Autodesk Inventor part; units mm, degrees
(part 3 of 3)
sketch "Sketch13" plane through (0, 0, 20) normal (0, 0, 1) x (1, 0, 0)
  arc A0 (68.9429, -68.9429) -> (69.4823, -68.3993) centre (0, 0) ccw projected
  arc A1 (69.4823, -68.3993) -> (73.8041, -70.4056) centre (83.4681, -43.9299) ccw projected
  arc A2 (73.8041, -70.4056) -> (74.9009, -69.2377) centre (0, 0) ccw projected
  arc A3 (74.9009, -69.2377) -> (72.6272, -65.0503) centre (49.0843, -80.5451) ccw projected
  arc A4 (72.6272, -65.0503) -> (73.64, -63.9015) centre (0, 0) ccw projected
  arc A5 (73.64, -63.9015) -> (78.0793, -65.6325) centre (86.0618, -38.6023) ccw projected
  arc A6 (78.0793, -65.6325) -> (79.1006, -64.398) centre (0, 0) ccw projected
  arc A7 (79.1006, -64.398) -> (76.5684, -60.3617) centre (54.0449, -77.3041) ccw projected
  arc A8 (76.5684, -60.3617) -> (77.5071, -59.1515) centre (0, 0) ccw projected
  arc A9 (77.5071, -59.1515) -> (82.0463, -60.6003) centre (88.3159, -33.1222) ccw projected
  arc A10 (82.0463, -60.6003) -> (82.9881, -59.3041) centre (0, 0) ccw projected
  arc A11 (82.9881, -59.3041) -> (80.2075, -55.4348) centre (58.7922, -73.758) ccw projected
  arc A12 (80.2075, -55.4348) -> (81.0683, -54.1681) centre (0, 0) ccw projected
  arc A13 (81.0683, -54.1681) -> (85.6895, -55.329) centre (90.2213, -27.5115) ccw projected
  arc A14 (85.6895, -55.329) -> (86.548, -53.9763) centre (0, 0) ccw projected
  arc A15 (86.548, -53.9763) -> (83.53, -50.2891) centre (63.3075, -69.9209) ccw projected
  arc A16 (83.53, -50.2891) -> (84.3096, -48.9709) centre (0, 0) ccw projected
  arc A17 (84.3096, -48.9709) -> (88.9946, -49.8394) centre (91.7708, -21.7921) ccw projected
  arc A18 (88.9946, -49.8394) -> (89.7665, -48.4354) centre (0, 0) ccw projected
  arc A19 (89.7665, -48.4354) -> (86.5228, -44.945) centre (67.5729, -65.8078) ccw projected
  arc A20 (86.5228, -44.945) -> (87.2181, -43.5804) centre (0, 0) ccw projected
  arc A21 (87.2181, -43.5804) -> (91.9484, -44.153) centre (92.958, -15.9868) ccw projected
  arc A22 (91.9484, -44.153) -> (92.6306, -42.7033) centre (0, 0) ccw projected
  arc A23 (92.6306, -42.7033) -> (89.1742, -39.4235) centre (71.5717, -61.435) ccw projected
  arc A24 (89.1742, -39.4235) -> (89.7824, -38.0179) centre (0, 0) ccw projected
  arc A25 (89.7824, -38.0179) -> (94.5394, -38.2924) centre (93.7784, -10.1184) ccw projected
  arc A26 (94.5394, -38.2924) -> (95.1292, -36.8027) centre (0, 0) ccw projected
  arc A27 (95.1292, -36.8027) -> (91.4737, -33.7464) centre (75.288, -56.8198) ccw projected
  arc A28 (91.4737, -33.7464) -> (91.9924, -32.3054) centre (0, 0) ccw projected
  arc A29 (91.9924, -32.3054) -> (96.7572, -32.2807) centre (94.2287, -4.21) ccw projected
  arc A30 (96.7572, -32.2807) -> (97.2523, -30.7569) centre (0, 0) ccw projected
  arc A31 (97.2523, -30.7569) -> (93.4121, -27.9361) centre (78.7072, -51.9803) ccw projected
  arc A32 (93.4121, -27.9361) -> (93.8394, -26.4654) centre (0, 0) ccw projected
  arc A33 (93.8394, -26.4654) -> (98.5932, -26.1415) centre (94.3071, 1.715) ccw projected
  arc A34 (98.5932, -26.1415) -> (98.9917, -24.5897) centre (0, 0) ccw projected
  arc A35 (98.9917, -24.5897) -> (94.9819, -22.0156) centre (81.8157, -46.9356) ccw projected
  arc A36 (94.9819, -22.0156) -> (95.316, -20.521) centre (0, 0) ccw projected
  arc A37 (95.316, -20.521) -> (100.0401, -19.8992) centre (94.0133, 7.6332) ccw projected
  arc A38 (100.0401, -19.8992) -> (100.3403, -18.3254) centre (0, 0) ccw projected
  arc A39 (100.3403, -18.3254) -> (96.1769, -16.0082) centre (84.6014, -41.7058) ccw projected
  arc A40 (96.1769, -16.0082) -> (96.4164, -14.4956) centre (0, 0) ccw projected
  arc A41 (96.4164, -14.4956) -> (101.0922, -13.5784) centre (93.3485, 13.5213) ccw projected
  arc A42 (101.0922, -13.5784) -> (101.293, -11.9888) centre (0, 0) ccw projected
  arc A43 (101.293, -11.9888) -> (96.9922, -9.9376) centre (87.0532, -36.3113) ccw projected
  arc A44 (96.9922, -9.9376) -> (97.1364, -8.4129) centre (0, 0) ccw projected
  arc A45 (97.1364, -8.4129) -> (101.7453, -7.204) centre (92.3153, 19.356) ccw projected
  arc A46 (101.7453, -7.204) -> (101.8459, -5.6049) centre (0, 0) ccw projected
  arc A47 (101.8459, -5.6049) -> (97.4248, -3.8278) centre (89.1614, -30.7735) ccw projected
  arc A48 (97.4248, -3.8278) -> (97.4729, -2.2971) centre (0, 0) ccw projected
  arc A49 (97.4729, -2.2971) -> (101.9969, -0.8011) centre (90.9178, 25.1143) ccw projected
  arc A50 (101.9969, -0.8011) -> (101.9969, 0.8011) centre (0, 0) ccw projected
  arc A51 (101.9969, 0.8011) -> (97.4729, 2.2971) centre (90.9178, -25.1143) ccw projected
  arc A52 (97.4729, 2.2971) -> (97.4248, 3.8278) centre (0, 0) ccw projected
  arc A53 (97.4248, 3.8278) -> (101.8459, 5.6049) centre (89.1614, 30.7735) ccw projected
  arc A54 (101.8459, 5.6049) -> (101.7453, 7.204) centre (0, 0) ccw projected
  arc A55 (101.7453, 7.204) -> (97.1364, 8.4129) centre (92.3153, -19.356) ccw projected
  arc A56 (97.1364, 8.4129) -> (96.9922, 9.9376) centre (0, 0) ccw projected
  arc A57 (96.9922, 9.9376) -> (101.293, 11.9888) centre (87.0532, 36.3113) ccw projected
  arc A58 (101.293, 11.9888) -> (101.0922, 13.5784) centre (0, 0) ccw projected
  arc A59 (101.0922, 13.5784) -> (96.4164, 14.4956) centre (93.3485, -13.5213) ccw projected
  arc A60 (96.4164, 14.4956) -> (96.1769, 16.0082) centre (0, 0) ccw projected
  arc A61 (96.1769, 16.0082) -> (100.3403, 18.3254) centre (84.6014, 41.7058) ccw projected
  arc A62 (100.3403, 18.3254) -> (100.0401, 19.8992) centre (0, 0) ccw projected
  arc A63 (100.0401, 19.8992) -> (95.316, 20.521) centre (94.0133, -7.6332) ccw projected
  arc A64 (95.316, 20.521) -> (94.9819, 22.0156) centre (0, 0) ccw projected
  arc A65 (94.9819, 22.0156) -> (98.9917, 24.5897) centre (81.8157, 46.9356) ccw projected
  arc A66 (98.9917, 24.5897) -> (98.5932, 26.1415) centre (0, 0) ccw projected
  arc A67 (98.5932, 26.1415) -> (93.8394, 26.4654) centre (94.3071, -1.715) ccw projected
  arc A68 (93.8394, 26.4654) -> (93.4121, 27.9361) centre (0, 0) ccw projected
  arc A69 (93.4121, 27.9361) -> (97.2523, 30.7569) centre (78.7072, 51.9803) ccw projected
  arc A70 (97.2523, 30.7569) -> (96.7572, 32.2807) centre (0, 0) ccw projected
  arc A71 (96.7572, 32.2807) -> (91.9924, 32.3054) centre (94.2287, 4.21) ccw projected
  arc A72 (91.9924, 32.3054) -> (91.4737, 33.7464) centre (0, 0) ccw projected
  arc A73 (91.4737, 33.7464) -> (95.1292, 36.8027) centre (75.288, 56.8198) ccw projected
  arc A74 (95.1292, 36.8027) -> (94.5394, 38.2924) centre (0, 0) ccw projected
  arc A75 (94.5394, 38.2924) -> (89.7824, 38.0179) centre (93.7784, 10.1184) ccw projected
  arc A76 (89.7824, 38.0179) -> (89.1742, 39.4235) centre (0, 0) ccw projected
  arc A77 (89.1742, 39.4235) -> (92.6306, 42.7033) centre (71.5717, 61.435) ccw projected
  arc A78 (92.6306, 42.7033) -> (91.9484, 44.153) centre (0, 0) ccw projected
  arc A79 (91.9484, 44.153) -> (87.2181, 43.5804) centre (92.958, 15.9868) ccw projected
  arc A80 (87.2181, 43.5804) -> (86.5228, 44.945) centre (0, 0) ccw projected
  arc A81 (86.5228, 44.945) -> (89.7665, 48.4354) centre (67.5729, 65.8078) ccw projected
  arc A82 (89.7665, 48.4354) -> (88.9946, 49.8394) centre (0, 0) ccw projected
  arc A83 (88.9946, 49.8394) -> (84.3096, 48.9709) centre (91.7708, 21.7921) ccw projected
  arc A84 (84.3096, 48.9709) -> (83.53, 50.2891) centre (0, 0) ccw projected
  arc A85 (83.53, 50.2891) -> (86.548, 53.9763) centre (63.3075, 69.9209) ccw projected
  arc A86 (86.548, 53.9763) -> (85.6895, 55.329) centre (0, 0) ccw projected
  arc A87 (85.6895, 55.329) -> (81.0683, 54.1681) centre (90.2213, 27.5115) ccw projected
  arc A88 (81.0683, 54.1681) -> (80.2075, 55.4348) centre (0, 0) ccw projected
  arc A89 (80.2075, 55.4348) -> (82.9881, 59.3041) centre (58.7922, 73.758) ccw projected
  arc A90 (82.9881, 59.3041) -> (82.0463, 60.6003) centre (0, 0) ccw projected
  arc A91 (82.0463, 60.6003) -> (77.5071, 59.1515) centre (88.3159, 33.1222) ccw projected
  arc A92 (77.5071, 59.1515) -> (76.5684, 60.3617) centre (0, 0) ccw projected
  arc A93 (76.5684, 60.3617) -> (79.1006, 64.398) centre (54.0449, 77.3041) ccw projected
  arc A94 (79.1006, 64.398) -> (78.0793, 65.6325) centre (0, 0) ccw projected
  arc A95 (78.0793, 65.6325) -> (73.64, 63.9015) centre (86.0618, 38.6023) ccw projected
  arc A96 (73.64, 63.9015) -> (72.6272, 65.0503) centre (0, 0) ccw projected
  arc A97 (72.6272, 65.0503) -> (74.9009, 69.2377) centre (49.0843, 80.5451) ccw projected
  arc A98 (74.9009, 69.2377) -> (73.8041, 70.4056) centre (0, 0) ccw projected
  arc A99 (73.8041, 70.4056) -> (69.4823, 68.3993) centre (83.4681, 43.9299) ccw projected
  arc A100 (69.4823, 68.3993) -> (68.3993, 69.4823) centre (0, 0) ccw projected
  arc A101 (68.3993, 69.4823) -> (70.4056, 73.8041) centre (43.9299, 83.4681) ccw projected
  arc A102 (70.4056, 73.8041) -> (69.2377, 74.9009) centre (0, 0) ccw projected
  arc A103 (69.2377, 74.9009) -> (65.0503, 72.6272) centre (80.5451, 49.0843) ccw projected
  arc A104 (65.0503, 72.6272) -> (63.9015, 73.64) centre (0, 0) ccw projected
  arc A105 (63.9015, 73.64) -> (65.6325, 78.0793) centre (38.6023, 86.0618) ccw projected
  arc A106 (65.6325, 78.0793) -> (64.398, 79.1006) centre (0, 0) ccw projected
  arc A107 (64.398, 79.1006) -> (60.3617, 76.5684) centre (77.3041, 54.0449) ccw projected
  arc A108 (60.3617, 76.5684) -> (59.1515, 77.5071) centre (0, 0) ccw projected
  arc A109 (59.1515, 77.5071) -> (60.6003, 82.0463) centre (33.1222, 88.3159) ccw projected
  arc A110 (60.6003, 82.0463) -> (59.3041, 82.9881) centre (0, 0) ccw projected
  arc A111 (59.3041, 82.9881) -> (55.4348, 80.2075) centre (73.758, 58.7922) ccw projected
  arc A112 (55.4348, 80.2075) -> (54.1681, 81.0683) centre (0, 0) ccw projected
  arc A113 (54.1681, 81.0683) -> (55.329, 85.6895) centre (27.5115, 90.2213) ccw projected
  arc A114 (55.329, 85.6895) -> (53.9763, 86.548) centre (0, 0) ccw projected
  arc A115 (53.9763, 86.548) -> (50.2891, 83.53) centre (69.9209, 63.3075) ccw projected
  arc A116 (50.2891, 83.53) -> (48.9709, 84.3096) centre (0, 0) ccw projected
  arc A117 (48.9709, 84.3096) -> (49.8394, 88.9946) centre (21.7921, 91.7708) ccw projected
  arc A118 (49.8394, 88.9946) -> (48.4354, 89.7665) centre (0, 0) ccw projected
  arc A119 (48.4354, 89.7665) -> (44.945, 86.5228) centre (65.8078, 67.5729) ccw projected
  arc A120 (44.945, 86.5228) -> (43.5804, 87.2181) centre (0, 0) ccw projected
  arc A121 (43.5804, 87.2181) -> (44.153, 91.9484) centre (15.9868, 92.958) ccw projected
  arc A122 (44.153, 91.9484) -> (42.7033, 92.6306) centre (0, 0) ccw projected
  arc A123 (42.7033, 92.6306) -> (39.4235, 89.1742) centre (61.435, 71.5717) ccw projected
  arc A124 (39.4235, 89.1742) -> (38.0179, 89.7824) centre (0, 0) ccw projected
  arc A125 (38.0179, 89.7824) -> (38.2924, 94.5394) centre (10.1184, 93.7784) ccw projected
  arc A126 (38.2924, 94.5394) -> (36.8027, 95.1292) centre (0, 0) ccw projected
  arc A127 (36.8027, 95.1292) -> (33.7464, 91.4737) centre (56.8198, 75.288) ccw projected
  arc A128 (33.7464, 91.4737) -> (32.3054, 91.9924) centre (0, 0) ccw projected
  arc A129 (32.3054, 91.9924) -> (32.2807, 96.7572) centre (4.21, 94.2287) ccw projected
  arc A130 (32.2807, 96.7572) -> (30.7569, 97.2523) centre (0, 0) ccw projected
  arc A131 (30.7569, 97.2523) -> (27.9361, 93.4121) centre (51.9803, 78.7072) ccw projected
  arc A132 (27.9361, 93.4121) -> (26.4654, 93.8394) centre (0, 0) ccw projected
  arc A133 (26.4654, 93.8394) -> (26.1415, 98.5932) centre (-1.715, 94.3071) ccw projected
  arc A134 (26.1415, 98.5932) -> (24.5897, 98.9917) centre (0, 0) ccw projected
  arc A135 (24.5897, 98.9917) -> (22.0156, 94.9819) centre (46.9356, 81.8157) ccw projected
  arc A136 (22.0156, 94.9819) -> (20.521, 95.316) centre (0, 0) ccw projected
  arc A137 (20.521, 95.316) -> (19.8992, 100.0401) centre (-7.6332, 94.0133) ccw projected
  arc A138 (19.8992, 100.0401) -> (18.3254, 100.3403) centre (0, 0) ccw projected
  arc A139 (18.3254, 100.3403) -> (16.0082, 96.1769) centre (41.7058, 84.6014) ccw projected
  arc A140 (16.0082, 96.1769) -> (14.4956, 96.4164) centre (0, 0) ccw projected
  arc A141 (14.4956, 96.4164) -> (13.5784, 101.0922) centre (-13.5213, 93.3485) ccw projected
  arc A142 (13.5784, 101.0922) -> (11.9888, 101.293) centre (0, 0) ccw projected
  arc A143 (11.9888, 101.293) -> (9.9376, 96.9922) centre (36.3113, 87.0532) ccw projected
  arc A144 (9.9376, 96.9922) -> (8.4129, 97.1364) centre (0, 0) ccw projected
  arc A145 (8.4129, 97.1364) -> (7.204, 101.7453) centre (-19.356, 92.3153) ccw projected
  arc A146 (7.204, 101.7453) -> (5.6049, 101.8459) centre (0, 0) ccw projected
  arc A147 (5.6049, 101.8459) -> (3.8278, 97.4248) centre (30.7735, 89.1614) ccw projected
  arc A148 (3.8278, 97.4248) -> (2.2971, 97.4729) centre (0, 0) ccw projected
  arc A149 (2.2971, 97.4729) -> (0.8011, 101.9969) centre (-25.1143, 90.9178) ccw projected
  arc A150 (0.8011, 101.9969) -> (-0.8011, 101.9969) centre (0, 0) ccw projected
  arc A151 (-0.8011, 101.9969) -> (-2.2971, 97.4729) centre (25.1143, 90.9178) ccw projected
  arc A152 (-2.2971, 97.4729) -> (-3.8278, 97.4248) centre (0, 0) ccw projected
  arc A153 (-3.8278, 97.4248) -> (-5.6049, 101.8459) centre (-30.7735, 89.1614) ccw projected
  arc A154 (-5.6049, 101.8459) -> (-7.204, 101.7453) centre (0, 0) ccw projected
  arc A155 (-7.204, 101.7453) -> (-8.4129, 97.1364) centre (19.356, 92.3153) ccw projected
  arc A156 (-8.4129, 97.1364) -> (-9.9376, 96.9922) centre (0, 0) ccw projected
  arc A157 (-9.9376, 96.9922) -> (-11.9888, 101.293) centre (-36.3113, 87.0532) ccw projected
  arc A158 (-11.9888, 101.293) -> (-13.5784, 101.0922) centre (0, 0) ccw projected
  arc A159 (-13.5784, 101.0922) -> (-14.4956, 96.4164) centre (13.5213, 93.3485) ccw projected
  arc A160 (-14.4956, 96.4164) -> (-16.0082, 96.1769) centre (0, 0) ccw projected
  arc A161 (-16.0082, 96.1769) -> (-18.3254, 100.3403) centre (-41.7058, 84.6014) ccw projected
  arc A162 (-18.3254, 100.3403) -> (-19.8992, 100.0401) centre (0, 0) ccw projected
  arc A163 (-19.8992, 100.0401) -> (-20.521, 95.316) centre (7.6332, 94.0133) ccw projected
  arc A164 (-20.521, 95.316) -> (-22.0156, 94.9819) centre (0, 0) ccw projected
  arc A165 (-22.0156, 94.9819) -> (-24.5897, 98.9917) centre (-46.9356, 81.8157) ccw projected
  arc A166 (-24.5897, 98.9917) -> (-26.1415, 98.5932) centre (0, 0) ccw projected
  arc A167 (-26.1415, 98.5932) -> (-26.4654, 93.8394) centre (1.715, 94.3071) ccw projected
  arc A168 (-26.4654, 93.8394) -> (-27.9361, 93.4121) centre (0, 0) ccw projected
  arc A169 (-27.9361, 93.4121) -> (-30.7569, 97.2523) centre (-51.9803, 78.7072) ccw projected
  arc A170 (-30.7569, 97.2523) -> (-32.2807, 96.7572) centre (0, 0) ccw projected
  arc A171 (-32.2807, 96.7572) -> (-32.3054, 91.9924) centre (-4.21, 94.2287) ccw projected
  arc A172 (-32.3054, 91.9924) -> (-33.7464, 91.4737) centre (0, 0) ccw projected
  arc A173 (-33.7464, 91.4737) -> (-36.8027, 95.1292) centre (-56.8198, 75.288) ccw projected
  arc A174 (-36.8027, 95.1292) -> (-38.2924, 94.5394) centre (0, 0) ccw projected
  arc A175 (-38.2924, 94.5394) -> (-38.0179, 89.7824) centre (-10.1184, 93.7784) ccw projected
  arc A176 (-38.0179, 89.7824) -> (-39.4235, 89.1742) centre (0, 0) ccw projected
  arc A177 (-39.4235, 89.1742) -> (-42.7033, 92.6306) centre (-61.435, 71.5717) ccw projected
  arc A178 (-42.7033, 92.6306) -> (-44.153, 91.9484) centre (0, 0) ccw projected
  arc A179 (-44.153, 91.9484) -> (-43.5804, 87.2181) centre (-15.9868, 92.958) ccw projected
  arc A180 (-43.5804, 87.2181) -> (-44.945, 86.5228) centre (0, 0) ccw projected
  arc A181 (-44.945, 86.5228) -> (-48.4354, 89.7665) centre (-65.8078, 67.5729) ccw projected
  arc A182 (-48.4354, 89.7665) -> (-49.8394, 88.9946) centre (0, 0) ccw projected
  arc A183 (-49.8394, 88.9946) -> (-48.9709, 84.3096) centre (-21.7921, 91.7708) ccw projected
  arc A184 (-48.9709, 84.3096) -> (-50.2891, 83.53) centre (0, 0) ccw projected
  arc A185 (-50.2891, 83.53) -> (-53.9763, 86.548) centre (-69.9209, 63.3075) ccw projected
  arc A186 (-53.9763, 86.548) -> (-55.329, 85.6895) centre (0, 0) ccw projected
  arc A187 (-55.329, 85.6895) -> (-54.1681, 81.0683) centre (-27.5115, 90.2213) ccw projected
  arc A188 (-54.1681, 81.0683) -> (-55.4348, 80.2075) centre (0, 0) ccw projected
  arc A189 (-55.4348, 80.2075) -> (-59.3041, 82.9881) centre (-73.758, 58.7922) ccw projected
  arc A190 (-59.3041, 82.9881) -> (-60.6003, 82.0463) centre (0, 0) ccw projected
  arc A191 (-60.6003, 82.0463) -> (-59.1515, 77.5071) centre (-33.1222, 88.3159) ccw projected
  arc A192 (-59.1515, 77.5071) -> (-60.3617, 76.5684) centre (0, 0) ccw projected
  arc A193 (-60.3617, 76.5684) -> (-64.398, 79.1006) centre (-77.3041, 54.0449) ccw projected
  arc A194 (-64.398, 79.1006) -> (-65.6325, 78.0793) centre (0, 0) ccw projected
  arc A195 (-65.6325, 78.0793) -> (-63.9015, 73.64) centre (-38.6023, 86.0618) ccw projected
  arc A196 (-63.9015, 73.64) -> (-65.0503, 72.6272) centre (0, 0) ccw projected
  arc A197 (-65.0503, 72.6272) -> (-69.2377, 74.9009) centre (-80.5451, 49.0843) ccw projected
  arc A198 (-69.2377, 74.9009) -> (-70.4056, 73.8041) centre (0, 0) ccw projected
  arc A199 (-70.4056, 73.8041) -> (-68.3993, 69.4823) centre (-43.9299, 83.4681) ccw projected
  arc A200 (-68.3993, 69.4823) -> (-68.9429, 68.9429) centre (0, 0) ccw projected
  line L0 (-68.9429, 68.9429) -> (-104.2983, 33.5876) projected
  line L1 (33.5876, -104.2983) -> (-104.2983, 33.5876) projected
  line L2 (68.9429, -68.9429) -> (33.5876, -104.2983) projected
  circle A201 centre (0, 0) radius 10 projected
  circle A202 centre (0, 0) radius 15
  dimension "d112" = 30
  constraints: 1 centre point, 1 coincident
  measures "d112" diameter of A202
extrude "Extrusion10" add sketch "Sketch13" along normal blind 15 contours A202
ref_plane "Work Plane11" through (-10.6066, -10.6066, 20) normal (-0.7071068, -0.7071068, 0) x (0.7071068, -0.7071068, 0)
sketch "Sketch14" plane through (-10.6066, -10.6066, 20) normal (-0.7071068, -0.7071068, 0) x (0.7071068, -0.7071068, 0)
  line L0 (15, 15) -> (-15, 15) projected
  line L1 (-15, 0) -> (15, 0) projected
  line L2 (-15, 0) -> (15, 0) projected
  line L3 (0, 0) -> (0, 15)
  circle A0 centre (0, 7.5) radius 3
  point P0 (0, -20)
  dimension "d115" = 6
  constraints: 3 midpoint, 2 end point, 1 centre point
  measures "d115" diameter of A0
extrude "Extrusion11" [suppressed]
thread "Thread4" size "M6x0.75" class "6H" standard "ANSI Metric M Profile" full length
chamfer "Chamfer1" distance 0.5 angle 45 2 edges at (-10, 0, 35) (7.0711, -7.0711, 0)
ref_plane "Work Plane12" through (0, 15, 20) normal (0, 1, 0) x (-1, 0, 0)
sketch "Sketch16" plane through (0, 15, 20) normal (0, 1, 0) x (-1, 0, 0)
  line L0 (15, 15) -> (-15, 15) projected
  line L1 (-15, 0) -> (15, 0) projected
  line L2 (15, 15) -> (-15, 15) projected
  line L3 (0, 15) -> (0, 0)
  circle A0 centre (0, 7.5) radius 3
  point P0 (0, -20)
  dimension "d123" = 6
  constraints: 3 midpoint, 2 end point, 1 centre point
  measures "d123" diameter of A0
extrude "Extrusion12" [suppressed]
thread "Thread5" size "M6x0.75" class "6H" standard "ANSI Metric M Profile" full length
ref_plane "Work Plane13" through (-15, 0, 20) normal (1, 0, 0) x (0, 1, 0)
sketch "Sketch17" plane through (-15, 0, 20) normal (1, 0, 0) x (0, 1, 0)
  line L0 (15, 15) -> (-15, 15) projected
  line L1 (-15, 0) -> (15, 0) projected
  line L2 (0, 0) -> (0, 15)
  line L3 (15, 15) -> (-15, 15) projected
  circle A0 centre (0, 7.5) radius 3
  point P0 (0, -20)
  dimension "d128" = 6
  constraints: 3 midpoint, 2 end point, 1 centre point
  measures "d128" diameter of A0
extrude "Extrusion13" [suppressed]
thread "Thread6" size "M6x0.75" class "6H" standard "ANSI Metric M Profile" full length
ref_plane "Work Plane14" through (15, 0, 20) normal (1, 0, 0) x (0, 1, 0)
sketch "Sketch18" plane through (15, 0, 20) normal (1, 0, 0) x (0, 1, 0)
  line L0 (15, 15) -> (-15, 15) projected
  line L1 (-15, 0) -> (15, 0) projected
  line L2 (0, 15) -> (0, 0)
  line L3 (-104.2983, 0) -> (33.5876, 0) projected
  circle A0 centre (0, 7.5) radius 3
  point P0 (0, -20)
  dimension "d133" = 6
  constraints: 2 end point, 2 midpoint, 1 centre point, 1 point on line, 1 vertical
  measures "d133" diameter of A0
extrude "Extrusion14" [suppressed]
thread "Thread7" size "M6x0.75" class "6H" standard "ANSI Metric M Profile" full length
ref_plane "Work Plane15" through (0, -15, 20) normal (0, 1, 0) x (-1, 0, 0)
sketch "Sketch19" plane through (0, -15, 20) normal (0, 1, 0) x (-1, 0, 0)
  line L0 (15, 15) -> (-15, 15) projected
  line L1 (-15, 0) -> (15, 0) projected
  line L2 (10.5, 15) -> (-10.5, 15) projected
  line L3 (0, 15) -> (0, 0)
  circle A0 centre (0, 7.5) radius 3
  point P0 (0, -20)
  dimension "d138" = 6
  constraints: 3 midpoint, 2 end point, 1 centre point
  measures "d138" diameter of A0
extrude "Extrusion15" cut sketch "Sketch19" along normal up to surface round surface about axis through (0, 0, 20) along (0, 0, -1) radius 10 far side no
thread "Thread8" size "M6x0.75" class "6H" standard "ANSI Metric M Profile" full length
sketch "Sketch20" plane through (0, 0, 20) normal (0, 0, 1) x (1, 0, 0)
  circle A0 centre (0, 0) radius 10 projected
  arc A1 (56.5685, -56.5685) -> (-56.5685, 56.5685) centre (0, 0) ccw
  line L0 (0, 0) -> (-56.5685, 56.5685)
  line L1 (-45.6084, 45.6084) -> (-49.851, 49.851) projected
  line L2 (0, 0) -> (56.5685, -56.5685)
  circle A2 centre (-56.5685, 56.5685) radius 0.5
  circle A3 centre (-55.5671, 57.5526) radius 0.5
  circle A4 centre (-54.5485, 58.5189) radius 0.5
  circle A5 centre (-53.5131, 59.4672) radius 0.5
  circle A6 centre (-52.4612, 60.3972) radius 0.5
  circle A7 centre (-51.3931, 61.3086) radius 0.5
  circle A8 centre (-50.3093, 62.2011) radius 0.5
  circle A9 centre (-49.2099, 63.0745) radius 0.5
  circle A10 centre (-48.0954, 63.9284) radius 0.5
  circle A11 centre (-46.966, 64.7626) radius 0.5
  circle A12 centre (-45.8222, 65.5769) radius 0.5
  circle A13 centre (-44.6643, 66.3709) radius 0.5
  circle A14 centre (-43.4926, 67.1446) radius 0.5
  circle A15 centre (-42.3075, 67.8975) radius 0.5
  circle A16 centre (-41.1094, 68.6296) radius 0.5
  circle A17 centre (-39.8986, 69.3405) radius 0.5
  circle A18 centre (-38.6756, 70.03) radius 0.5
  circle A19 centre (-37.4406, 70.698) radius 0.5
  circle A20 centre (-36.1941, 71.3442) radius 0.5
  circle A21 centre (-34.9364, 71.9684) radius 0.5
  circle A22 centre (-33.668, 72.5704) radius 0.5
  circle A23 centre (-32.3892, 73.1501) radius 0.5
  circle A24 centre (-31.1005, 73.7073) radius 0.5
  circle A25 centre (-29.8021, 74.2417) radius 0.5
  circle A26 centre (-28.4946, 74.7533) radius 0.5
  circle A27 centre (-27.1783, 75.2419) radius 0.5
  circle A28 centre (-25.8536, 75.7073) radius 0.5
  circle A29 centre (-24.521, 76.1493) radius 0.5
  circle A30 centre (-23.1808, 76.568) radius 0.5
  circle A31 centre (-21.8335, 76.963) radius 0.5
  circle A32 centre (-20.4794, 77.3343) radius 0.5
  circle A33 centre (-19.119, 77.6818) radius 0.5
  circle A34 centre (-17.7528, 78.0054) radius 0.5
  circle A35 centre (-16.3811, 78.3049) radius 0.5
  circle A36 centre (-15.0043, 78.5803) radius 0.5
  circle A37 centre (-13.6229, 78.8316) radius 0.5
  circle A38 centre (-12.2373, 79.0585) radius 0.5
  circle A39 centre (-10.848, 79.2611) radius 0.5
  circle A40 centre (-9.4553, 79.4393) radius 0.5
  circle A41 centre (-8.0597, 79.593) radius 0.5
  circle A42 centre (-6.6616, 79.7222) radius 0.5
  circle A43 centre (-5.2614, 79.8268) radius 0.5
  circle A44 centre (-3.8597, 79.9068) radius 0.5
  circle A45 centre (-2.4567, 79.9623) radius 0.5
  circle A46 centre (-1.053, 79.9931) radius 0.5
  circle A47 centre (0.351, 79.9992) radius 0.5
  circle A48 centre (1.7549, 79.9807) radius 0.5
  circle A49 centre (3.1583, 79.9376) radius 0.5
  circle A50 centre (4.5607, 79.8699) radius 0.5
  circle A51 centre (5.9617, 79.7776) radius 0.5
  circle A52 centre (7.3609, 79.6606) radius 0.5
  circle A53 centre (8.7578, 79.5192) radius 0.5
  circle A54 centre (10.152, 79.3532) radius 0.5
  circle A55 centre (11.5431, 79.1629) radius 0.5
  circle A56 centre (12.9306, 78.9481) radius 0.5
  circle A57 centre (14.3142, 78.709) radius 0.5
  circle A58 centre (15.6933, 78.4457) radius 0.5
  circle A59 centre (17.0676, 78.1582) radius 0.5
  circle A60 centre (18.4366, 77.8466) radius 0.5
  circle A61 centre (19.8, 77.511) radius 0.5
  circle A62 centre (21.1572, 77.1516) radius 0.5
  circle A63 centre (22.508, 76.7684) radius 0.5
  circle A64 centre (23.8518, 76.3616) radius 0.5
  circle A65 centre (25.1883, 75.9312) radius 0.5
  circle A66 centre (26.517, 75.4775) radius 0.5
  circle A67 centre (27.8375, 75.0005) radius 0.5
  circle A68 centre (29.1495, 74.5004) radius 0.5
  circle A69 centre (30.4525, 73.9773) radius 0.5
  circle A70 centre (31.7461, 73.4315) radius 0.5
  circle A71 centre (33.0299, 72.8631) radius 0.5
  circle A72 centre (34.3035, 72.2722) radius 0.5
  circle A73 centre (35.5666, 71.659) radius 0.5
  circle A74 centre (36.8188, 71.0238) radius 0.5
  circle A75 centre (38.0595, 70.3667) radius 0.5
  circle A76 centre (39.2886, 69.6879) radius 0.5
  circle A77 centre (40.5056, 68.9877) radius 0.5
  circle A78 centre (41.7101, 68.2662) radius 0.5
  circle A79 centre (42.9017, 67.5237) radius 0.5
  circle A80 centre (44.0801, 66.7603) radius 0.5
  circle A81 centre (45.245, 65.9765) radius 0.5
  circle A82 centre (46.3959, 65.1722) radius 0.5
  circle A83 centre (47.5325, 64.348) radius 0.5
  circle A84 centre (48.6545, 63.5039) radius 0.5
  circle A85 centre (49.7615, 62.6402) radius 0.5
  circle A86 centre (50.8531, 61.7572) radius 0.5
  circle A87 centre (51.9291, 60.8553) radius 0.5
  circle A88 centre (52.9892, 59.9345) radius 0.5
  circle A89 centre (54.0328, 58.9954) radius 0.5
  circle A90 centre (55.0599, 58.038) radius 0.5
  circle A91 centre (56.07, 57.0628) radius 0.5
  circle A92 centre (57.0628, 56.07) radius 0.5
  circle A93 centre (58.038, 55.0599) radius 0.5
  circle A94 centre (58.9954, 54.0328) radius 0.5
  circle A95 centre (59.9345, 52.9892) radius 0.5
  circle A96 centre (60.8553, 51.9291) radius 0.5
  circle A97 centre (61.7572, 50.8531) radius 0.5
  circle A98 centre (62.6402, 49.7615) radius 0.5
  circle A99 centre (63.5039, 48.6545) radius 0.5
  circle A100 centre (64.348, 47.5325) radius 0.5
  circle A101 centre (65.1722, 46.3959) radius 0.5
  circle A102 centre (65.9765, 45.245) radius 0.5
  circle A103 centre (66.7603, 44.0801) radius 0.5
  circle A104 centre (67.5237, 42.9017) radius 0.5
  circle A105 centre (68.2662, 41.7101) radius 0.5
  circle A106 centre (68.9877, 40.5056) radius 0.5
  circle A107 centre (69.6879, 39.2886) radius 0.5
  circle A108 centre (70.3667, 38.0595) radius 0.5
  circle A109 centre (71.0238, 36.8188) radius 0.5
  circle A110 centre (71.659, 35.5666) radius 0.5
  circle A111 centre (72.2722, 34.3035) radius 0.5
  circle A112 centre (72.8631, 33.0299) radius 0.5
  circle A113 centre (73.4315, 31.7461) radius 0.5
  circle A114 centre (73.9773, 30.4525) radius 0.5
  circle A115 centre (74.5004, 29.1495) radius 0.5
  circle A116 centre (75.0005, 27.8375) radius 0.5
  circle A117 centre (75.4775, 26.517) radius 0.5
  circle A118 centre (75.9312, 25.1883) radius 0.5
  circle A119 centre (76.3616, 23.8518) radius 0.5
  circle A120 centre (76.7684, 22.508) radius 0.5
  circle A121 centre (77.1516, 21.1572) radius 0.5
  circle A122 centre (77.511, 19.8) radius 0.5
  circle A123 centre (77.8466, 18.4366) radius 0.5
  circle A124 centre (78.1582, 17.0676) radius 0.5
  circle A125 centre (78.4457, 15.6933) radius 0.5
  circle A126 centre (78.709, 14.3142) radius 0.5
  circle A127 centre (78.9481, 12.9306) radius 0.5
  circle A128 centre (79.1629, 11.5431) radius 0.5
  circle A129 centre (79.3532, 10.152) radius 0.5
  circle A130 centre (79.5192, 8.7578) radius 0.5
  circle A131 centre (79.6606, 7.3609) radius 0.5
  circle A132 centre (79.7776, 5.9617) radius 0.5
  circle A133 centre (79.8699, 4.5607) radius 0.5
  circle A134 centre (79.9376, 3.1583) radius 0.5
  circle A135 centre (79.9807, 1.7549) radius 0.5
  circle A136 centre (79.9992, 0.351) radius 0.5
  circle A137 centre (79.9931, -1.053) radius 0.5
  circle A138 centre (79.9623, -2.4567) radius 0.5
  circle A139 centre (79.9068, -3.8597) radius 0.5
  circle A140 centre (79.8268, -5.2614) radius 0.5
  circle A141 centre (79.7222, -6.6616) radius 0.5
  circle A142 centre (79.593, -8.0597) radius 0.5
  circle A143 centre (79.4393, -9.4553) radius 0.5
  circle A144 centre (79.2611, -10.848) radius 0.5
  circle A145 centre (79.0585, -12.2373) radius 0.5
  circle A146 centre (78.8316, -13.6229) radius 0.5
  circle A147 centre (78.5803, -15.0043) radius 0.5
  circle A148 centre (78.3049, -16.3811) radius 0.5
  circle A149 centre (78.0054, -17.7528) radius 0.5
  circle A150 centre (77.6818, -19.119) radius 0.5
  circle A151 centre (77.3343, -20.4794) radius 0.5
  circle A152 centre (76.963, -21.8335) radius 0.5
  circle A153 centre (76.568, -23.1808) radius 0.5
  circle A154 centre (76.1493, -24.521) radius 0.5
  circle A155 centre (75.7073, -25.8536) radius 0.5
  circle A156 centre (75.2419, -27.1783) radius 0.5
  circle A157 centre (74.7533, -28.4946) radius 0.5
  circle A158 centre (74.2417, -29.8021) radius 0.5
  circle A159 centre (73.7073, -31.1005) radius 0.5
  circle A160 centre (73.1501, -32.3892) radius 0.5
  circle A161 centre (72.5704, -33.668) radius 0.5
  circle A162 centre (71.9684, -34.9364) radius 0.5
  circle A163 centre (71.3442, -36.1941) radius 0.5
  circle A164 centre (70.698, -37.4406) radius 0.5
  circle A165 centre (70.03, -38.6756) radius 0.5
  circle A166 centre (69.3405, -39.8986) radius 0.5
  circle A167 centre (68.6296, -41.1094) radius 0.5
  circle A168 centre (67.8975, -42.3075) radius 0.5
  circle A169 centre (67.1446, -43.4926) radius 0.5
  circle A170 centre (66.3709, -44.6643) radius 0.5
  circle A171 centre (65.5769, -45.8222) radius 0.5
  circle A172 centre (64.7626, -46.966) radius 0.5
  circle A173 centre (63.9284, -48.0954) radius 0.5
  circle A174 centre (63.0745, -49.2099) radius 0.5
  circle A175 centre (62.2011, -50.3093) radius 0.5
  circle A176 centre (61.3086, -51.3931) radius 0.5
  circle A177 centre (60.3972, -52.4612) radius 0.5
  circle A178 centre (59.4672, -53.5131) radius 0.5
  circle A179 centre (58.5189, -54.5485) radius 0.5
  circle A180 centre (57.5526, -55.5671) radius 0.5
  circle A181 centre (56.5685, -56.5685) radius 0.5
  dimension "d143" = 160
  dimension "d144" = 1
  dimension "d147" = 180
  constraints: 181 centre point, 4 end point, 2 coincident, 2 point on circle, 1 collinear, 359 other
  measures "d143" diameter of A1
  measures "d144" diameter of A2
sketch "Sketch25" plane through (0, 0, 20) normal (0, 0, 1) x (1, 0, 0)
  circle A0 centre (0, 0) radius 15 projected
  line L0 (0, 0) -> (38.8909, 38.8909)
  line L1 (0, 0) -> (55, 0) construction
  circle A1 centre (0, 0) radius 10 projected
  circle A2 centre (0, 0) radius 25
  arc A3 (28.5554, -63.9108) -> (-63.9108, 28.5554) centre (0, 0) ccw
  line L2 (0, 0) -> (-35.3553, -35.3553)
  line L3 (-104.2983, 33.5876) -> (33.5876, -104.2983) projected
  line L4 (0, 0) -> (50, 0) construction
  line L5 (-17.6777, -17.6777) -> (51.2652, -86.6206)
  line L6 (68.9429, -68.9429) -> (33.5876, -104.2983) projected
  line L7 (-17.6777, -17.6777) -> (79.8223, -17.6777) construction
  line L8 (-17.6777, -17.6777) -> (-86.6206, 51.2652)
  line L9 (-68.9429, 68.9429) -> (-104.2983, 33.5876) projected
  line L10 (-17.6777, -17.6777) -> (79.8223, -17.6777) construction
  dimension "d178" = 45
  dimension "d180" = 140
  dimension "d181" = 135
  dimension "d182" = 45
  dimension "d183" = 135
  constraints: 16 end point, 4 equal length, 4 horizontal, 4 midpoint, 3 coincident, 2 point on circle, 2 point on line, 1 centre point, 3 other
  measures "d178" angle of L1 L0
  measures "d180" diameter of A3
  measures "d181" angle of L2 L4
  measures "d182" angle of L5 L7
  measures "d183" angle of L10 L8
sketch "Sketch26" plane through (-56.5685, -14.1421, 20) normal (-0.7071068, -0.7071068, 0) x (0, 0, -1)
  line L0 (203, 102) -> (203, 0)
  line L1 (0, 102) -> (203, 102)
  line L2 (0, 0) -> (0, 102)
  line L3 (0, 0) -> (203, 0)
  circle A0 centre (10, -8.1) radius 4.2
  circle A1 centre (10, 12.5) radius 4.2
  circle A2 centre (10, 47.5) radius 4.2
  circle A3 centre (10, 68.1) radius 4.2
  line L4 (10, 12.5) -> (10, 47.5)
  circle A4 centre (10, 30) radius 3.5 projected
  line L5 (10, 30) -> (-0.5049, 30)
  circle A5 centre (10, 68.1) radius 4
  circle A6 centre (10, 47.5) radius 4
  circle A7 centre (10, 12.5) radius 4
  circle A8 centre (10, -8.1) radius 4
  point P0 (20, 30)
  dimension "d203" = 8
  dimension "d204" = 8
  dimension "d205" = 8
  dimension "d206" = 8
  constraints: 12 end point, 8 centre point, 4 coincident, 1 midpoint
  measures "d203" diameter of A5
  measures "d204" diameter of A6
  measures "d205" diameter of A7
  measures "d206" diameter of A8
ref_plane "Work Plane16" through (-14.1421, -14.1421, 10) normal (-0.7071068, -0.7071068, 0) x (-0.7071068, 0.7071068, 0)
ref_plane "Work Plane17" through (-14.1421, -14.1421, 10) normal (-0.7071068, -0.7071068, 0) x (-0.7071068, 0.7071068, 0)
ref_plane "Work Plane19" through (47.7297, -47.7297, 10) normal (-0.7071068, -0.7071068, 0) x (-0.7071068, 0.7071068, 0)
ref_plane "Work Plane20" through (-47.7297, 47.7297, 10) normal (-0.7071068, -0.7071068, 0) x (-0.7071068, 0.7071068, 0)
ref_plane "Work Plane22" through (-47.7297, 47.7297, 10) normal (-0.7071068, -0.7071068, 0) x (-0.7071068, 0.7071068, 0)
extrude "Extrusion16" cut sketch "Sketch26" against normal blind 50 contours A5 | A6 | A7 | A8
ref_plane "Work Plane24" through (-14.1421, -14.1421, 10) normal (-0.7071068, -0.7071068, 0) x (-0.7071068, 0.7071068, 0)
ref_plane "Work Plane25" through (47.7297, -47.7297, 10) normal (-0.7071068, -0.7071068, 0) x (-0.7071068, 0.7071068, 0)
thread "Thread13" size "M8x1.25" class "6H" standard "ANSI Metric M Profile" full length
thread "Thread14" size "M8x1.25" class "6H" standard "ANSI Metric M Profile" full length
thread "Thread15" size "M8x1.25" class "6H" standard "ANSI Metric M Profile" full length
thread "Thread16" size "M8x1.25" class "6H" standard "ANSI Metric M Profile" full length
chamfer "Chamfer5" distance 0.7 angle 45 4 edges at (-8.4146, -62.2961, 14) (-22.981, -47.7297, 14) (-47.7297, -22.981, 14) (-62.2961, -8.4146, 14)
sketch "Sketch9" plane through (-14.1421, -14.1421, 10) normal (-0.7071068, -0.7071068, 0) x (-0.7071068, 0.7071068, 0)
  point P0 (0, 0)
sketch "Sketch10" plane through (47.7297, -47.7297, 10) normal (-0.7071068, -0.7071068, 0) x (-0.7071068, 0.7071068, 0)
  point P0 (0, 0)
sketch "Sketch11" plane through (-47.7297, 47.7297, 10) normal (-0.7071068, -0.7071068, 0) x (-0.7071068, 0.7071068, 0)
  point P0 (0, 0)
sketch "Sketch21" plane through (-14.1421, -14.1421, 10) normal (-0.7071068, -0.7071068, 0) x (-0.7071068, 0.7071068, 0)
  point P0 (0, 0)
sketch "Sketch22" plane through (-14.1421, -14.1421, 10) normal (-0.7071068, -0.7071068, 0) x (-0.7071068, 0.7071068, 0)
  point P0 (0, 0)
sketch "Sketch23" plane through (47.7297, -47.7297, 10) normal (-0.7071068, -0.7071068, 0) x (-0.7071068, 0.7071068, 0)
  point P0 (0, 0)
sketch "Sketch24" plane through (-47.7297, 47.7297, 10) normal (-0.7071068, -0.7071068, 0) x (-0.7071068, 0.7071068, 0)
  point P0 (0, 0)
sketch "Sketch27" plane through (-26.9408, 26.9408, 10) normal (-0.7071068, -0.7071068, 0) x (-0.7071068, 0.7071068, 0)
  point P0 (0, 0)
hole "Hole12" at (-26.9408, 26.9408, 10) direction (0.7071068, 0.7071068, 0) diameter 6.647 depth 5 tip angle 120 thread size "M8x1.25" class "6H" standard "ISO Metric profile"
sketch "Sketch28" plane through (-12.3744, 12.3744, 10) normal (-0.7071068, -0.7071068, 0) x (-0.7071068, 0.7071068, 0)
  point P0 (0, 0)
hole "Hole14" at (-12.3744, 12.3744, 10) direction (0.7071068, 0.7071068, 0) diameter 6.647 depth 5 tip angle 120 thread size "M8x1.25" class "6H" standard "ISO Metric profile"
sketch "Sketch30" plane through (12.3744, -12.3744, 10) normal (-0.7071068, -0.7071068, 0) x (-0.7071068, 0.7071068, 0)
  point P0 (0, 0)
hole "Hole17" at (12.3744, -12.3744, 10) direction (0.7071068, 0.7071068, 0) diameter 6.647 depth 5 tip angle 120 thread size "M8x1.25" class "6H" standard "ISO Metric profile"
sketch "Sketch31" plane through (26.9408, -26.9408, 10) normal (-0.7071068, -0.7071068, 0) x (-0.7071068, 0.7071068, 0)
  point P0 (0, 0)
hole "Hole19" at (26.9408, -26.9408, 10) direction (0.7071068, 0.7071068, 0) diameter 6.647 depth 5 tip angle 120 thread size "M8x1.25" class "6H" standard "ISO Metric profile"
equation "\"d0\" = da_da"
equation "\"d1\" = da_b"
equation "\"d3\" = da_dw"
equation "\"da_da\" = 204"
equation "\"da_b\" = 20"
equation "\"da_dw\" = 200"
body "Solid1"
body "Srf1"
